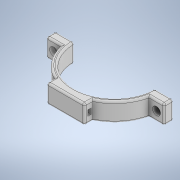
# Autodesk Inventor part: ur5e_cable_tube_top_85mm
Saved by Autodesk Inventor 2020 (Build 240168000, 168)
## iProperties
Created: 2021-03-04
Part Number: ur5e_cable_tube_top_85mm
Material: Generic
Document SubType Name: Modeling
Designer: NILY
Density: 1 g/cm^3
Appearance: Default
Author: NILY
Autodesk Inventor part; units mm, degrees
ref_plane "XZ Plane" through (0, 0, 0) normal (0, 1, 0) x (-1, 0, 0)
sketch "Sketch1" plane through (0, 0, 0) normal (0, 1, 0) x (-1, 0, 0)
  circle A0 centre (0, 0) radius 47.5
  dimension "d0" = 95
  constraints: 1 centre point, 1 coincident
  measures "d0" diameter of A0
extrude "Extrusion1" add sketch "Sketch1" along normal blind 20
shell "Shell1" thickness 5 removed faces 2 at (-10.3648, 20, 5.7529) at (-10.3648, 0, 5.7529)
sketch "Sketch2" plane through (0, 20, 0) normal (0, 1, 0) x (1, 0, 0)
  line L0 (-62.0625, 51.3519) -> (57.6609, 51.3519)
  line L1 (57.6609, 51.3519) -> (57.6609, 0)
  line L2 (57.6609, 0) -> (-62.0625, 0)
  line L3 (-62.0625, 0) -> (-62.0625, 51.3519)
  point P0 (0, 0)
  constraints: 8 end point, 2 parallel, 1 horizontal, 1 perpendicular
extrude "Extrusion2" cut sketch "Sketch2" against normal through all
ref_plane "Work Plane1" through (-47.5, 0, 0) normal (1, 0, 0) x (0, 1, 0)
sketch "Sketch3" plane through (-47.5, 0, 0) normal (1, 0, 0) x (0, 1, 0)
  line L0 (0, 0) -> (0, 47.5) projected
  line L1 (0, 0) -> (20, 0)
  line L2 (20, 0) -> (20, 10)
  line L3 (20, 10) -> (0, 10)
  line L4 (0, 10) -> (0, 0)
  point P0 (0, 10)
  dimension "d7" = 20
  dimension "d8" = 10
  constraints: 8 end point, 2 parallel, 1 horizontal, 1 perpendicular
  measures "d7" distance of L3.end L2.end
  measures "d8" distance of L2.end L1.end
extrude "Extrusion3" add sketch "Sketch3" along normal blind 2 and the other way blind 15
mirror "Mirror1" about plane through (0, 0, 0) normal (1, 0, 0) of "Extrusion3"
sketch "Sketch5" plane through (-62.5, 20, 10) normal (0, 0, 1) x (1, 0, 0)
  line L0 (0, -20) -> (0, 0) projected
  line L1 (0, 0) -> (16.0646, 0) projected
  point P0 (62.5, -20)
  point P1 (8.0323, -10)
  point P2 (0, -10)
  point P3 (8.0323, 0)
  constraints: 2 midpoint, 1 horizontal alignment, 1 vertical alignment
hole "Hole2" at (-54.4677, 10, 10) direction (0, 0, -1) diameter 5.5 end through all counterbore diameter 8.5 counterbore depth 5 clearance for "Hex Head Bolt" size "M5" standard "Ansi Metric M Profile"
mirror "Mirror2" about plane through (0, 0, 0) normal (1, 0, 0) of "Hole2"
ref_plane "Work Plane2" through (0, 0, 45) normal (0, 0, 1) x (1, 0, 0)
sketch "Sketch6" plane through (0, 0, 45) normal (0, 0, 1) x (1, 0, 0)
  line L0 (46.4354, 20) -> (-46.4354, 20) projected
  line L1 (42.5, 0) -> (-42.5, 0) projected
  line L2 (-20, 20) -> (20, 20)
  line L3 (20, 20) -> (20, 0)
  line L4 (20, 0) -> (-20, 0)
  line L5 (-20, 0) -> (-20, 20)
  point P0 (0, 0)
  point P1 (0, 20)
  point P2 (0, 20)
  dimension "d28" = 40
  constraints: 8 end point, 2 midpoint, 2 parallel, 2 point on line, 1 coincident, 1 horizontal, 1 perpendicular
  measures "d28" distance of L3.end L4.end
extrude "Extrusion4" add sketch "Sketch6" along normal blind 7 and the other way blind 2.5
fillet "Fillet1" radius 2 32 edges at (0, 0, 42.5) (-37.1087, 0, 29.6512) (-20, 0, 47.5421) (-20, 10, 52) (0, 0, 52) (20, 10, 52) (20, 0, 47.5421) (0, 20, 42.5) (37.1087, 0, 29.6512) (37.1087, 20, 29.6512) (54.4677, 0, 10) (-52.5, 0, 0) (52.5, 0, 0) (62.5, 0, 5) (62.5, 20, 5) (62.5, 10, 0) (62.5, 10, 10) (54.4677, 20, 10) (-52.5, 20, 0) (52.5, 20, 0) (-42.5, 10, 0) (42.5, 10, 0) (0, 20, 52) (20, 20, 47.5421) (-20, 20, 47.5421) (-37.1087, 20, 29.6512) (-54.4677, 20, 10) (-62.5, 20, 5) (-62.5, 10, 0) (-62.5, 10, 10) (-62.5, 0, 5) (-54.4677, 0, 10)
sketch "Sketch10" plane through (-20, 2, 43.0842) normal (-1, 0, 0) x (0, 0, 1)
  line L0 (4.7079, 10.5) -> (2.2079, 10.5)
  line L1 (2.2079, 10.5) -> (2.2079, 5.5)
  line L2 (2.2079, 5.5) -> (4.7079, 5.5)
  line L3 (4.7079, 5.5) -> (4.7079, 10.5)
  line L4 (6.9158, 16) -> (6.9158, 0) projected
  line L5 (0, 16) -> (6.9158, 16) projected
  point P0 (-43.0842, -2)
  point P1 (4.7079, 8)
  point P2 (6.9158, 8)
  point P3 (3.4579, 10.5)
  point P4 (3.4579, 16)
  dimension "d43" = 2.5
  dimension "d44" = 5
  constraints: 8 end point, 4 midpoint, 2 parallel, 1 horizontal, 1 horizontal alignment, 1 perpendicular, 1 vertical alignment
  measures "d43" distance of L2.end L1.end
  measures "d44" distance of L1.end L0.end
extrude "Extrusion6" cut sketch "Sketch10" against normal through all
chamfer "Chamfer2" distance 0.5 angle 45 8 edges at (-20, 10, 47.7921) (-20, 12.5, 46.5421) (-20, 10, 45.2921) (-20, 7.5, 46.5421) (20, 7.5, 46.5421) (20, 10, 47.7921) (20, 10, 45.2921) (20, 12.5, 46.5421)
body "Solid1"
